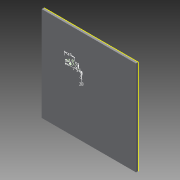
# Autodesk Inventor part: lcdgen
Saved by Autodesk Inventor 2014 (Build 180170000, 170)
## iProperties
Created: 2015-05-09
Part Number: lcdgen
Material: Generic
Document SubType Name: Modeling
Designer: cruiser
Density: 1 g/cm^3
Appearance: Default
Author: cruiser
Autodesk Inventor part; units mm, degrees
ref_plane "YZ Plane" through (0, 0, 0) normal (1, 0, 0) x (0, 1, 0)
ref_plane "XZ Plane" through (0, 0, 0) normal (0, 1, 0) x (-1, 0, 0)
ref_plane "XY Plane" through (0, 0, 0) normal (0, 0, 1) x (1, 0, 0)
sketch "Sketch3" plane through (0, 0, 0) normal (0, 1, 0) x (-1, 0, 0)
  line L0 (200, -200) -> (-200, -200)
  line L1 (-200, -200) -> (-200, 200)
  line L2 (-200, 200) -> (200, 200)
  line L3 (200, 200) -> (200, -200)
  line L4 (200, -200) -> (-200, 200) construction
  line L5 (-200, -200) -> (200, 200) construction
  point P0 (0, 0)
  dimension "d8" = 400
  dimension "d9" = 400
  constraints: 12 end point, 2 midpoint, 2 parallel, 1 horizontal, 1 perpendicular
  measures "d8" distance of L1.end L2.end
  measures "d9" distance of L0.end L1.end
extrude "Extrusion1" add sketch "Sketch3" along normal blind 10
sketch "Sketch1" plane through (0, 10, 0) normal (0, 1, 0) x (1, 0, 0)
  line L0 (-110.207, -17.8784) -> (-36.207, -17.8784)
  line L1 (-36.207, -17.8784) -> (-36.207, -45.8784)
  line L2 (-36.207, -45.8784) -> (-110.207, -45.8784)
  line L3 (-110.207, -45.8784) -> (-110.207, -17.8784)
  line L4 (-114.707, -49.9784) -> (-69.707, -49.9784)
  line L5 (-69.707, -49.9784) -> (-69.707, -66.9784)
  line L6 (-69.707, -66.9784) -> (-114.707, -66.9784)
  line L7 (-114.707, -66.9784) -> (-114.707, -49.9784)
  line L8 (-114.707, -58.4784) -> (-69.707, -58.4784)
  line L9 (200, 200) -> (-200, 200) projected
  line L10 (-200, 200) -> (-200, -200) projected
  line L11 (-200, -200) -> (200, -200) projected
  line L12 (200, -200) -> (200, 200) projected
  point P0 (0, 0)
  dimension "d2" = 74
  dimension "d3" = 28
  dimension "d4" = 45
  dimension "d5" = 17
  dimension "d6" = 12.6
  dimension "d7" = 40.5
  constraints: 18 end point, 4 parallel, 2 horizontal, 2 midpoint, 2 perpendicular
  measures "d2" distance of L1.end L2.end
  measures "d3" distance of L0.end L1.end
  measures "d4" distance of L5.end L6.end
  measures "d5" distance of L4.end L5.end
  measures "d6" distance between parallel lines of L2 L8
  measures "d7" distance between parallel lines of L5 L3
body "Solid1"
